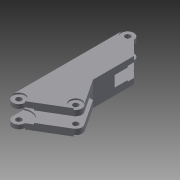
# Autodesk Inventor part: Pinky_Lower_main_1
Saved by Autodesk Inventor 2015 (Build 190159000, 159)
## iProperties
Created: 2016-07-08
Part Number: Pinky_Lower_main_1
Material: Generic
Document SubType Name: Modeling
Designer: Neelotpal Nag
Density: 1 g/cm^3
Appearance: Default
Author: Neelotpal Nag
Autodesk Inventor part; units mm, degrees
ref_plane "YZ Plane" through (0, 0, 0) normal (1, 0, 0) x (0, 1, 0)
sketch "Sketch1" plane through (0, 0, 0) normal (0, 0, 1) x (1, 0, 0)
  circle A0 centre (0, 0) radius 1
  circle A1 centre (0, 0) radius 2.25
  circle A2 centre (0, 40) radius 1
  circle A3 centre (0, 40) radius 2.25
  line L0 (-2.25, 40) -> (-2.25, 0)
  line L1 (0, 0) -> (15, 0) construction
  line L2 (12.2873, 8.6036) -> (11.2873, 8.6036)
  circle A4 centre (12.2873, 8.6036) radius 1
  circle A5 centre (12.2873, 8.6036) radius 2.25
  line L3 (2.25, 0) -> (13.4395, 6.671)
  line L4 (2.25, 40) -> (7.9069, 34.3431)
  line L5 (7.9069, 34.3431) -> (7.9069, 19.3431)
  line L6 (7.9069, 19.3431) -> (14.1662, 9.8414)
  line L7 (0, 0) -> (0, 1)
  line L8 (0, 39) -> (0, 40)
  line L9 (0, 0) -> (1.8431, 1.2905)
  line L10 (11.4681, 8.0301) -> (12.2873, 8.6036)
  dimension "d5" = 2
  dimension "d7" = 2
  dimension "d0" = 40
  dimension "d6" = 4.5
  dimension "d8" = 4.5
  dimension "d9" = 15
  dimension "d11" = 2
  dimension "d12" = 4.5
  dimension "d13" = 8
  dimension "d15" = 15
  constraints: 22 end point, 9 point on circle, 6 coincident, 4 centre point, 3 tangent, 3 vertical, 2 parallel, 2 perpendicular, 2 vertical alignment, 1 horizontal, 1 point on line, 4 other
  measures "d0" distance of L7.start L8.end
  measures "d6" diameter of A1
  measures "d8" diameter of A3
  measures "d9" distance of L1.start L2.start
  measures "d11" diameter of A4
  measures "d12" diameter of A5
  measures "d13" distance of L4.start L4.end
  measures "d15" distance of L4.end L5.end
ref_plane "Work Plane1" through (0, 0, 2) normal (0, 0, 1) x (1, 0, 0)
extrude "Extrusion1" add sketch "Sketch1" against normal blind 2.5 contours A1 L0 A3 L4 L5 L6 A5 L3
extrude "Extrusion2" add sketch "Sketch1" against normal blind 2 contours A1 | A5 | A3
mirror "Mirror1" about plane through (0, 0, 2) normal (0, 0, 1) of "Extrusion1", "Extrusion2"
sketch "Sketch2" plane through (0, 0, 0) normal (0, 0, 1) x (1, 0, 0)
  line L0 (0, 37.5855) -> (-2.2556, 37.5855)
  line L1 (-2.2556, 37.5855) -> (-2.2556, 29.5855)
  line L2 (-2.2556, 29.5855) -> (0, 29.5855)
  line L3 (0, 29.5855) -> (0, 37.5855)
  point P0 (0, 0)
  dimension "d21" = 8
  constraints: 8 end point, 2 perpendicular, 1 horizontal, 1 vertical
  measures "d21" distance of L0.end L1.end
extrude "Extrusion3" add sketch "Sketch2" along normal blind 6
sketch "Sketch3" plane through (0, 0, 6.5) normal (0, 0, 1) x (1, 0, 0)
  line L0 (7.9069, 19.3431) -> (5.9069, 19.3431)
  line L1 (5.9069, 19.3431) -> (5.9069, 27.3431)
  line L2 (5.9069, 27.3431) -> (7.9069, 27.3431)
  line L3 (7.9069, 27.3431) -> (7.9069, 19.3431)
  point P0 (0, 0)
  dimension "d24" = 2
  dimension "d25" = 8
  constraints: 8 end point, 2 parallel, 1 horizontal, 1 perpendicular
  measures "d24" distance of L1.end L2.end
  measures "d25" distance of L0.end L1.end
extrude "Extrusion4" add sketch "Sketch3" against normal blind 9
sketch "Sketch6" plane through (0, 0, 4) normal (0, 0, -1) x (-1, 0, 0)
  circle A0 centre (0, 0) radius 4.5
  dimension "d33" = 9
  constraints: 1 centre point, 1 coincident
  measures "d33" diameter of A0
extrude "Extrusion7" cut sketch "Sketch6" against normal blind 0.5
sketch "Sketch7" plane through (0, 0, 0) normal (0, 0, 1) x (1, 0, 0)
  circle A0 centre (0, 0) radius 4.5
  dimension "d36" = 9
  constraints: 1 centre point, 1 coincident
  measures "d36" diameter of A0
extrude "Extrusion8" cut sketch "Sketch7" against normal blind 0.5
sketch "Sketch8" plane through (0, 40, 4) normal (0, 0, -1) x (-1, 0, 0)
  circle A0 centre (0, 0) radius 2.5
  line L0 (-1.7678, -1.7678) -> (-6.7819, -6.7819)
  circle A1 centre (0, 0) radius 2.5
  line L1 (-7.9069, -5.6569) -> (-2.4944, -0.2556)
  arc A2 (-2.4876, -0.2488) -> (-1.7678, -1.7678) centre (0, 0) ccw
  arc A3 (-2.4876, -0.2488) -> (-1.7678, -1.7678) centre (0, 0) ccw
  line L2 (-7.9069, -5.6569) -> (-2.4876, -0.2488)
  line L3 (-7.9069, -5.6569) -> (-7.9069, -7.9069)
  line L4 (-6.7819, -6.7819) -> (-7.9069, -7.9069)
  point P0 (0, -40)
  dimension "d39" = 5
  constraints: 10 end point, 4 point on circle, 3 centre point, 3 coincident, 1 collinear, 1 vertical, 4 other
  measures "d39" diameter of A0
extrude "Extrusion9" cut sketch "Sketch8" against normal blind 0.5
ref_plane "Work Plane2" through (0, 0, 2) normal (0, 0, -1) x (-1, 0, 0)
mirror "Mirror2" about plane through (0, 0, 2) normal (0, 0, -1) of "Extrusion9"
body "Solid1"
